Autodesk Inventor part; units mm, degrees
(part 2 of 2)
sketch "Sketch10" plane through (0, 5.08, 0) normal (0, 1, 0) x (1, 0, 0)
  line L0 (-146.4702, 23.2181) -> (-107.0908, 23.2181) construction
  line L1 (-107.0908, 23.2181) -> (-107.0908, 13.5732) construction
  line L2 (-107.0908, 13.5732) -> (-146.4702, 13.5732) construction
  line L3 (-146.4702, 13.5732) -> (-146.4702, 23.2181) construction
  spline S0 degree 2 poles (-138.3409, 21.7608) (-138.5381, 21.3498) (-139.1463, 19.9801) knots 0 0 0 1 1 1
  spline S1 degree 2 poles (-139.1463, 19.9801) (-139.6503, 18.8296) (-140.001, 18.1776) knots 0 0 0 1 1 1
  spline S2 degree 2 poles (-140.001, 18.1776) (-140.6146, 17.0489) (-140.6584, 16.9777) knots 0 0 0 1 1 1
  spline S3 degree 2 poles (-140.6584, 16.9777) (-140.8886, 16.638) (-141.1899, 16.638) knots 0 0 0 1 1 1
  spline S4 degree 2 poles (-141.1899, 16.638) (-141.409, 16.638) (-141.5734, 16.7805) knots 0 0 0 1 1 1
  spline S5 degree 2 poles (-141.5734, 16.7805) (-141.7542, 16.9394) (-141.7542, 17.1695) knots 0 0 0 1 1 1
  spline S6 degree 2 poles (-141.7542, 17.1695) (-141.7542, 17.3612) (-140.9324, 18.7857) knots 0 0 0 1 1 1
  spline S7 degree 2 poles (-140.9324, 18.7857) (-141.2337, 19.224) (-141.798, 20.1116) knots 0 0 0 1 1 1
  spline S8 degree 2 poles (-141.798, 20.1116) (-142.2254, 20.7636) (-143.0472, 22.0785) knots 0 0 0 1 1 1
  spline S9 degree 2 poles (-143.0472, 22.0785) (-143.1239, 22.2155) (-143.1239, 22.358) knots 0 0 0 1 1 1
  spline S10 degree 2 poles (-143.1239, 22.358) (-143.1239, 22.5881) (-142.9486, 22.7415) knots 0 0 0 1 1 1
  spline S11 degree 2 poles (-142.9486, 22.7415) (-142.7788, 22.8894) (-142.5596, 22.8894) knots 0 0 0 1 1 1
  spline S12 degree 2 poles (-142.5596, 22.8894) (-142.3021, 22.8894) (-142.0884, 22.6264) knots 0 0 0 1 1 1
  line L4 (-142.0884, 22.6264) -> (-141.7926, 22.1552)
  spline S13 degree 2 poles (-141.7926, 22.1552) (-141.7652, 22.1059) (-141.1187, 21.0047) knots 0 0 0 1 1 1
  spline S14 degree 2 poles (-141.1187, 21.0047) (-140.7132, 20.3034) (-140.4009, 19.8979) knots 0 0 0 1 1 1
  spline S15 degree 2 poles (-140.4009, 19.8979) (-140.0996, 20.4951) (-139.5408, 21.7169) knots 0 0 0 1 1 1
  spline S16 degree 2 poles (-139.5408, 21.7169) (-139.4202, 21.9854) (-139.1846, 22.5333) knots 0 0 0 1 1 1
  spline S17 degree 2 poles (-139.1846, 22.5333) (-139.0367, 22.8894) (-138.6751, 22.8894) knots 0 0 0 1 1 1
  spline S18 degree 2 poles (-138.6751, 22.8894) (-138.4559, 22.8894) (-138.2916, 22.747) knots 0 0 0 1 1 1
  spline S19 degree 2 poles (-138.2916, 22.747) (-138.1108, 22.5935) (-138.1108, 22.3634) knots 0 0 0 1 1 1
  spline S20 degree 2 poles (-138.1108, 22.3634) (-138.1108, 22.2319) (-138.3409, 21.7608) knots 0 0 0 1 1 1
  spline S21 degree 2 poles (-133.6126, 21.9525) (-133.6893, 21.9525) (-133.777, 21.9744) knots 0 0 0 1 1 1
  spline S22 degree 2 poles (-133.777, 21.9744) (-134.4125, 22.1443) (-135.0152, 22.1443) knots 0 0 0 1 1 1
  spline S23 degree 2 poles (-135.0152, 22.1443) (-135.3111, 22.1443) (-135.985, 22.0511) (-136.3685, 21.958) knots 0 0 0 1 2 2 2
  spline S24 degree 2 poles (-136.3685, 21.958) (-136.3685, 21.4375) (-136.4014, 20.4075) knots 0 0 0 1 1 1
  spline S25 degree 2 poles (-136.4014, 20.4075) (-136.1822, 20.4239) (-134.8618, 20.5499) knots 0 0 0 1 1 1
  spline S26 degree 2 poles (-134.8618, 20.5499) (-134.1112, 20.6266) (-133.914, 20.6266) knots 0 0 0 1 1 1
  spline S27 degree 2 poles (-133.914, 20.6266) (-133.6784, 20.6266) (-133.3496, 20.3308) (-133.3496, 20.0897) knots 0 0 0 1 2 2 2
  spline S28 degree 2 poles (-133.3496, 20.0897) (-133.3496, 19.6185) (-133.8482, 19.5583) knots 0 0 0 1 1 1
  spline S29 degree 2 poles (-133.8482, 19.5583) (-134.166, 19.5363) (-134.7906, 19.4816) knots 0 0 0 1 1 1
  spline S30 degree 2 poles (-134.7906, 19.4816) (-135.3494, 19.4158) (-136.4726, 19.3281) knots 0 0 0 1 1 1
  spline S31 degree 2 poles (-136.4726, 19.3281) (-136.5, 18.8296) (-136.5, 18.5228) knots 0 0 0 1 1 1
  spline S32 degree 2 poles (-136.5, 18.5228) (-136.5, 17.7448) (-136.4123, 17.6407) knots 0 0 0 1 1 1
  spline S33 degree 2 poles (-136.4123, 17.6407) (-136.3685, 17.5913) (-135.9137, 17.5913) knots 0 0 0 1 1 1
  spline S34 degree 2 poles (-135.9137, 17.5913) (-135.6727, 17.5913) (-134.6865, 17.6133) (-134.4399, 17.6133) knots 0 0 0 1 2 2 2
  spline S35 degree 2 poles (-134.4399, 17.6133) (-134.3632, 17.6133) (-134.0564, 17.6626) (-133.9797, 17.6626) knots 0 0 0 1 2 2 2
  spline S36 degree 2 poles (-133.9797, 17.6626) (-133.7496, 17.6626) (-133.5907, 17.5311) knots 0 0 0 1 1 1
  spline S37 degree 2 poles (-133.5907, 17.5311) (-133.4044, 17.3832) (-133.4044, 17.1256) knots 0 0 0 1 1 1
  spline S38 degree 2 poles (-133.4044, 17.1256) (-133.4044, 16.6819) (-133.8647, 16.5997) knots 0 0 0 1 1 1
  spline S39 degree 2 poles (-133.8647, 16.5997) (-134.2591, 16.523) (-135.4974, 16.523) knots 0 0 0 1 1 1
  spline S40 degree 2 poles (-135.4974, 16.523) (-136.7794, 16.523) (-137.1684, 16.8681) knots 0 0 0 1 1 1
  spline S41 degree 2 poles (-137.1684, 16.8681) (-137.5958, 17.2517) (-137.5958, 18.5228) knots 0 0 0 1 1 1
  spline S42 degree 2 poles (-137.5958, 18.5228) (-137.5958, 19.0487) (-137.4478, 21.1581) (-137.4478, 21.6786) knots 0 0 0 1 2 2 2
  spline S43 degree 2 poles (-137.4478, 21.6786) (-137.4478, 21.821) (-137.5245, 22.358) (-137.5245, 22.4949) knots 0 0 0 1 2 2 2
  spline S44 degree 2 poles (-137.5245, 22.4949) (-137.5245, 23.0921) (-136.9766, 23.0921) knots 0 0 0 1 1 1
  spline S45 degree 2 poles (-136.9766, 23.0921) (-136.8013, 23.0921) (-136.6589, 22.9935) knots 0 0 0 1 1 1
  spline S46 degree 2 poles (-136.6589, 22.9935) (-136.1987, 23.1086) (-135.3823, 23.2181) (-135.0152, 23.2181) knots 0 0 0 1 2 2 2
  spline S47 degree 2 poles (-135.0152, 23.2181) (-134.0235, 23.2181) (-133.4318, 22.9935) knots 0 0 0 1 1 1
  spline S48 degree 2 poles (-133.4318, 22.9935) (-133.0702, 22.8565) (-133.0702, 22.4949) knots 0 0 0 1 1 1
  spline S49 degree 2 poles (-133.0702, 22.4949) (-133.0702, 22.2922) (-133.2127, 22.1333) knots 0 0 0 1 1 1
  spline S50 degree 2 poles (-133.2127, 22.1333) (-133.3716, 21.9525) (-133.6126, 21.9525) knots 0 0 0 1 1 1
  spline S51 degree 2 poles (-130.6979, 16.6709) (-131.695, 16.6709) (-132.2703, 17.1147) knots 0 0 0 1 1 1
  spline S52 degree 2 poles (-132.2703, 17.1147) (-132.7524, 17.4818) (-132.7524, 17.9639) knots 0 0 0 1 1 1
  spline S53 degree 2 poles (-132.7524, 17.9639) (-132.7524, 18.2159) (-132.4566, 18.5392) (-132.1936, 18.5392) knots 0 0 0 1 2 2 2
  spline S54 degree 2 poles (-132.1936, 18.5392) (-131.8375, 18.5392) (-131.6731, 18.1776) knots 0 0 0 1 1 1
  spline S55 degree 2 poles (-131.6731, 18.1776) (-131.4485, 17.6954) (-130.6595, 17.6954) knots 0 0 0 1 1 1
  spline S56 degree 2 poles (-130.6595, 17.6954) (-129.9801, 17.6954) (-129.3501, 17.9913) knots 0 0 0 1 1 1
  spline S57 degree 2 poles (-129.3501, 17.9913) (-128.6926, 18.2926) (-128.6926, 18.6542) knots 0 0 0 1 1 1
  spline S58 degree 2 poles (-128.6926, 18.6542) (-128.6926, 19.1528) (-129.1035, 19.3117) knots 0 0 0 1 1 1
  spline S59 degree 2 poles (-129.1035, 19.3117) (-129.3939, 19.4213) (-130.2705, 19.4432) knots 0 0 0 1 1 1
  spline S60 degree 2 poles (-130.2705, 19.4432) (-130.9499, 19.4596) (-131.4868, 19.7007) knots 0 0 0 1 1 1
  spline S61 degree 2 poles (-131.4868, 19.7007) (-132.2155, 20.024) (-132.2046, 20.6321) knots 0 0 0 1 1 1
  spline S62 degree 2 poles (-132.2046, 20.6321) (-132.1936, 21.3992) (-130.5828, 22.6757) (-129.6076, 22.6757) knots 0 0 0 1 2 2 2
  spline S63 degree 2 poles (-129.6076, 22.6757) (-129.2241, 22.6757) (-128.6543, 22.5004) knots 0 0 0 1 1 1
  spline S64 degree 2 poles (-128.6543, 22.5004) (-127.953, 22.2813) (-127.953, 21.9909) knots 0 0 0 1 1 1
  spline S65 degree 2 poles (-127.953, 21.9909) (-127.953, 21.7882) (-128.0954, 21.6293) knots 0 0 0 1 1 1
  spline S66 degree 2 poles (-128.0954, 21.6293) (-128.2543, 21.4539) (-128.5009, 21.4539) knots 0 0 0 1 1 1
  spline S67 degree 2 poles (-128.5009, 21.4539) (-128.6817, 21.4539) (-129.4213, 21.6128) (-129.6076, 21.6128) knots 0 0 0 1 2 2 2
  spline S68 degree 2 poles (-129.6076, 21.6128) (-130.1171, 21.6074) (-130.5719, 21.3718) knots 0 0 0 1 1 1
  spline S69 degree 2 poles (-130.5719, 21.3718) (-131.043, 21.1252) (-131.043, 20.8403) knots 0 0 0 1 1 1
  spline S70 degree 2 poles (-131.043, 20.8403) (-131.043, 20.6869) (-130.7581, 20.4951) (-130.4678, 20.4568) knots 0 0 0 1 2 2 2
  spline S71 degree 2 poles (-130.4678, 20.4568) (-129.9692, 20.4294) (-129.4651, 20.402) knots 0 0 0 1 1 1
  spline S72 degree 2 poles (-129.4651, 20.402) (-128.594, 20.3363) (-128.0899, 19.9089) knots 0 0 0 1 1 1
  spline S73 degree 2 poles (-128.0899, 19.9089) (-127.5311, 19.4377) (-127.5311, 18.6049) knots 0 0 0 1 1 1
  spline S74 degree 2 poles (-127.5311, 18.6049) (-127.5311, 17.5913) (-128.6871, 17.0654) knots 0 0 0 1 1 1
  spline S75 degree 2 poles (-128.6871, 17.0654) (-129.5638, 16.6709) (-130.6979, 16.6709) knots 0 0 0 1 1 1
  spline S76 degree 2 poles (-115.8063, 21.9525) (-115.8721, 21.7936) (-115.9652, 21.558) knots 0 0 0 1 1 1
  spline S77 degree 2 poles (-115.9652, 21.558) (-116.031, 21.3279) (-116.1789, 20.8841) knots 0 0 0 1 1 1
  spline S78 degree 2 poles (-116.1789, 20.8841) (-116.4035, 20.3034) (-116.8911, 19.1967) knots 0 0 0 1 1 1
  spline S79 degree 2 poles (-116.8911, 19.1967) (-117.3897, 18.0735) (-117.6089, 17.5201) knots 0 0 0 1 1 1
  spline S80 degree 2 poles (-117.6089, 17.5201) (-117.7678, 17.1092) (-117.9102, 16.8627) knots 0 0 0 1 1 1
  spline S81 degree 2 poles (-117.9102, 16.8627) (-118.0965, 16.5339) (-118.4745, 16.5339) knots 0 0 0 1 1 1
  spline S82 degree 2 poles (-118.4745, 16.5339) (-118.6937, 16.5339) (-118.8745, 16.6545) knots 0 0 0 1 1 1
  spline S83 degree 2 poles (-118.8745, 16.6545) (-119.0882, 16.7969) (-119.1046, 17.027) knots 0 0 0 1 1 1
  spline S84 degree 2 poles (-119.1046, 17.027) (-119.2854, 17.4818) (-119.3347, 17.7667) knots 0 0 0 1 1 1
  spline S85 degree 2 poles (-119.3347, 17.7667) (-119.5046, 18.6104) (-119.8114, 20.2979) knots 0 0 0 1 1 1
  spline S86 degree 2 poles (-119.8114, 20.2979) (-120.0689, 19.5035) (-120.3647, 18.8789) knots 0 0 0 1 1 1
  spline S87 degree 2 poles (-120.3647, 18.8789) (-120.8031, 17.931) (-120.94, 17.3941) knots 0 0 0 1 1 1
  spline S88 degree 2 poles (-120.94, 17.3941) (-120.9071, 17.3064) (-120.9071, 17.2078) knots 0 0 0 1 1 1
  spline S89 degree 2 poles (-120.9071, 17.2078) (-120.9071, 16.9668) (-121.1208, 16.8133) knots 0 0 0 1 1 1
  spline S90 degree 2 poles (-121.1208, 16.8133) (-121.3126, 16.6819) (-121.5372, 16.6819) knots 0 0 0 1 1 1
  spline S91 degree 2 poles (-121.5372, 16.6819) (-121.8276, 16.6819) (-122.0139, 16.8298) knots 0 0 0 1 1 1
  spline S92 degree 2 poles (-122.0139, 16.8298) (-122.2221, 16.9887) (-122.2276, 17.2681) knots 0 0 0 1 1 1
  line L5 (-122.2276, 17.2681) -> (-122.3481, 17.7283)
  spline S93 degree 2 poles (-122.3481, 17.7283) (-122.4796, 18.342) (-122.7754, 19.5583) knots 0 0 0 1 1 1
  spline S94 degree 2 poles (-122.7754, 19.5583) (-123.0329, 20.4951) (-123.6466, 22.2155) knots 0 0 0 1 1 1
  spline S95 degree 2 poles (-123.6466, 22.2155) (-123.6795, 22.3141) (-123.6795, 22.4127) knots 0 0 0 1 1 1
  spline S96 degree 2 poles (-123.6795, 22.4127) (-123.6795, 22.6483) (-123.4987, 22.7853) knots 0 0 0 1 1 1
  spline S97 degree 2 poles (-123.4987, 22.7853) (-123.3398, 22.9113) (-123.1097, 22.9113) knots 0 0 0 1 1 1
  spline S98 degree 2 poles (-123.1097, 22.9113) (-122.8083, 22.9113) (-122.633, 22.6593) knots 0 0 0 1 1 1
  spline S99 degree 2 poles (-122.633, 22.6593) (-122.5344, 22.5223) (-122.4084, 22.1607) knots 0 0 0 1 1 1
  spline S100 degree 2 poles (-122.4084, 22.1607) (-122.0248, 21.0485) (-121.5372, 18.9282) knots 0 0 0 1 1 1
  spline S101 degree 2 poles (-121.5372, 18.9282) (-121.2249, 19.6952) (-120.8962, 20.7362) knots 0 0 0 1 1 1
  spline S102 degree 2 poles (-120.8962, 20.7362) (-120.6332, 21.5854) (-120.4688, 21.947) knots 0 0 0 1 1 1
  spline S103 degree 2 poles (-120.4688, 21.947) (-120.0744, 22.8017) (-119.6689, 22.8017) knots 0 0 0 1 1 1
  spline S104 degree 2 poles (-119.6689, 22.8017) (-119.2799, 22.8017) (-119.1046, 22.3799) knots 0 0 0 1 1 1
  spline S105 degree 2 poles (-119.1046, 22.3799) (-119.0169, 22.1826) (-118.9348, 21.6512) knots 0 0 0 1 1 1
  spline S106 degree 2 poles (-118.9348, 21.6512) (-118.9128, 21.4923) (-118.8361, 20.8622) knots 0 0 0 1 1 1
  spline S107 degree 2 poles (-118.8361, 20.8622) (-118.7485, 20.1883) (-118.3376, 18.4022) knots 0 0 0 1 1 1
  spline S108 degree 2 poles (-118.3376, 18.4022) (-117.9212, 19.3775) (-117.2199, 21.2129) knots 0 0 0 1 1 1
  spline S109 degree 2 poles (-117.2199, 21.2129) (-117.176, 21.3225) (-117.0117, 21.9361) knots 0 0 0 1 1 1
  spline S110 degree 2 poles (-117.0117, 21.9361) (-116.9021, 22.3744) (-116.7268, 22.6319) knots 0 0 0 1 1 1
  spline S111 degree 2 poles (-116.7268, 22.6319) (-116.5405, 22.9058) (-116.2227, 22.9058) knots 0 0 0 1 1 1
  spline S112 degree 2 poles (-116.2227, 22.9058) (-115.9817, 22.9058) (-115.6694, 22.61) (-115.6694, 22.3799) knots 0 0 0 1 2 2 2
  spline S113 degree 2 poles (-115.6694, 22.3799) (-115.6694, 22.2977) (-115.8063, 21.9525) knots 0 0 0 1 1 1
  spline S114 degree 2 poles (-111.1493, 21.9525) (-111.226, 21.9525) (-111.3137, 21.9744) knots 0 0 0 1 1 1
  spline S115 degree 2 poles (-111.3137, 21.9744) (-111.9492, 22.1443) (-112.5519, 22.1443) knots 0 0 0 1 1 1
  spline S116 degree 2 poles (-112.5519, 22.1443) (-112.8477, 22.1443) (-113.5216, 22.0511) (-113.9052, 21.958) knots 0 0 0 1 2 2 2
  spline S117 degree 2 poles (-113.9052, 21.958) (-113.9052, 21.4375) (-113.938, 20.4075) knots 0 0 0 1 1 1
  spline S118 degree 2 poles (-113.938, 20.4075) (-113.7189, 20.4239) (-112.3985, 20.5499) knots 0 0 0 1 1 1
  spline S119 degree 2 poles (-112.3985, 20.5499) (-111.6479, 20.6266) (-111.4506, 20.6266) knots 0 0 0 1 1 1
  spline S120 degree 2 poles (-111.4506, 20.6266) (-111.215, 20.6266) (-110.8863, 20.3308) (-110.8863, 20.0897) knots 0 0 0 1 2 2 2
  spline S121 degree 2 poles (-110.8863, 20.0897) (-110.8863, 19.6185) (-111.3849, 19.5583) knots 0 0 0 1 1 1
  spline S122 degree 2 poles (-111.3849, 19.5583) (-111.7027, 19.5363) (-112.3273, 19.4816) knots 0 0 0 1 1 1
  spline S123 degree 2 poles (-112.3273, 19.4816) (-112.8861, 19.4158) (-114.0093, 19.3281) knots 0 0 0 1 1 1
  spline S124 degree 2 poles (-114.0093, 19.3281) (-114.0367, 18.8296) (-114.0367, 18.5228) knots 0 0 0 1 1 1
  spline S125 degree 2 poles (-114.0367, 18.5228) (-114.0367, 17.7448) (-113.949, 17.6407) knots 0 0 0 1 1 1
  spline S126 degree 2 poles (-113.949, 17.6407) (-113.9052, 17.5913) (-113.4504, 17.5913) knots 0 0 0 1 1 1
  spline S127 degree 2 poles (-113.4504, 17.5913) (-113.2093, 17.5913) (-112.2232, 17.6133) (-111.9766, 17.6133) knots 0 0 0 1 2 2 2
  spline S128 degree 2 poles (-111.9766, 17.6133) (-111.8999, 17.6133) (-111.5931, 17.6626) (-111.5164, 17.6626) knots 0 0 0 1 2 2 2
  spline S129 degree 2 poles (-111.5164, 17.6626) (-111.2863, 17.6626) (-111.1274, 17.5311) knots 0 0 0 1 1 1
  spline S130 degree 2 poles (-111.1274, 17.5311) (-110.9411, 17.3832) (-110.9411, 17.1256) knots 0 0 0 1 1 1
  spline S131 degree 2 poles (-110.9411, 17.1256) (-110.9411, 16.6819) (-111.4013, 16.5997) knots 0 0 0 1 1 1
  spline S132 degree 2 poles (-111.4013, 16.5997) (-111.7958, 16.523) (-113.034, 16.523) knots 0 0 0 1 1 1
  spline S133 degree 2 poles (-113.034, 16.523) (-114.3161, 16.523) (-114.7051, 16.8681) knots 0 0 0 1 1 1
  spline S134 degree 2 poles (-114.7051, 16.8681) (-115.1324, 17.2517) (-115.1324, 18.5228) knots 0 0 0 1 1 1
  spline S135 degree 2 poles (-115.1324, 18.5228) (-115.1324, 19.0487) (-114.9845, 21.1581) (-114.9845, 21.6786) knots 0 0 0 1 2 2 2
  spline S136 degree 2 poles (-114.9845, 21.6786) (-114.9845, 21.821) (-115.0612, 22.358) (-115.0612, 22.4949) knots 0 0 0 1 2 2 2
  spline S137 degree 2 poles (-115.0612, 22.4949) (-115.0612, 23.0921) (-114.5133, 23.0921) knots 0 0 0 1 1 1
  spline S138 degree 2 poles (-114.5133, 23.0921) (-114.338, 23.0921) (-114.1955, 22.9935) knots 0 0 0 1 1 1
  spline S139 degree 2 poles (-114.1955, 22.9935) (-113.7353, 23.1086) (-112.919, 23.2181) (-112.5519, 23.2181) knots 0 0 0 1 2 2 2
  spline S140 degree 2 poles (-112.5519, 23.2181) (-111.5602, 23.2181) (-110.9685, 22.9935) knots 0 0 0 1 1 1
  spline S141 degree 2 poles (-110.9685, 22.9935) (-110.6069, 22.8565) (-110.6069, 22.4949) knots 0 0 0 1 1 1
  spline S142 degree 2 poles (-110.6069, 22.4949) (-110.6069, 22.2922) (-110.7493, 22.1333) knots 0 0 0 1 1 1
  spline S143 degree 2 poles (-110.7493, 22.1333) (-110.9082, 21.9525) (-111.1493, 21.9525) knots 0 0 0 1 1 1
  spline S144 degree 2 poles (-134.4153, 7.617) (-134.7659, 7.617) (-134.9358, 7.9896) knots 0 0 0 1 1 1
  spline S145 degree 2 poles (-134.9358, 7.9896) (-135.0125, 8.1704) (-135.0947, 8.2033) knots 0 0 0 1 1 1
  spline S146 degree 2 poles (-135.0947, 8.2033) (-135.1549, 8.2307) (-135.407, 8.2307) knots 0 0 0 1 1 1
  spline S147 degree 2 poles (-135.407, 8.2307) (-135.9001, 8.2307) (-136.5466, 7.4581) knots 0 0 0 1 1 1
  spline S148 degree 2 poles (-136.5466, 7.4581) (-137.456, 6.3843) (-137.456, 5.4419) knots 0 0 0 1 1 1
  spline S149 degree 2 poles (-137.456, 5.4419) (-137.456, 5.0146) (-136.8808, 4.4009) (-136.4808, 4.4009) knots 0 0 0 1 2 2 2
  spline S150 degree 2 poles (-136.4808, 4.4009) (-136.0918, 4.4009) (-135.6919, 4.6037) knots 0 0 0 1 1 1
  spline S151 degree 2 poles (-135.6919, 4.6037) (-135.5494, 4.6804) (-135.0947, 4.9927) knots 0 0 0 1 1 1
  spline S152 degree 2 poles (-135.0947, 4.9927) (-134.7878, 5.1954) (-134.629, 5.1954) knots 0 0 0 1 1 1
  spline S153 degree 2 poles (-134.629, 5.1954) (-134.3934, 5.1954) (-134.229, 5.0201) knots 0 0 0 1 1 1
  spline S154 degree 2 poles (-134.229, 5.0201) (-134.0756, 4.8612) (-134.0756, 4.653) knots 0 0 0 1 1 1
  spline S155 degree 2 poles (-134.0756, 4.653) (-134.0756, 4.4229) (-134.2783, 4.2475) knots 0 0 0 1 1 1
  spline S156 degree 2 poles (-134.2783, 4.2475) (-135.3631, 3.338) (-136.4808, 3.338) knots 0 0 0 1 1 1
  spline S157 degree 2 poles (-136.4808, 3.338) (-137.3684, 3.338) (-137.9765, 3.9845) knots 0 0 0 1 1 1
  spline S158 degree 2 poles (-137.9765, 3.9845) (-138.5573, 4.6037) (-138.5573, 5.4419) knots 0 0 0 1 1 1
  spline S159 degree 2 poles (-138.5573, 5.4419) (-138.5573, 6.7623) (-137.4067, 8.132) knots 0 0 0 1 1 1
  spline S160 degree 2 poles (-137.4067, 8.132) (-136.426, 9.2936) (-135.407, 9.2936) knots 0 0 0 1 1 1
  spline S161 degree 2 poles (-135.407, 9.2936) (-135.2316, 9.2936) (-134.9522, 9.2716) (-134.8481, 9.2443) knots 0 0 0 1 2 2 2
  spline S162 degree 2 poles (-134.8481, 9.2443) (-134.6728, 9.4141) (-134.4317, 9.4141) knots 0 0 0 1 1 1
  spline S163 degree 2 poles (-134.4317, 9.4141) (-134.0263, 9.4141) (-133.9331, 8.9539) knots 0 0 0 1 1 1
  spline S164 degree 2 poles (-133.9331, 8.9539) (-133.8674, 8.6251) (-133.8674, 8.1868) knots 0 0 0 1 1 1
  spline S165 degree 2 poles (-133.8674, 8.1868) (-133.8674, 7.9896) (-133.9825, 7.8307) knots 0 0 0 1 1 1
  spline S166 degree 2 poles (-133.9825, 7.8307) (-134.1304, 7.617) (-134.4153, 7.617) knots 0 0 0 1 1 1
  spline S167 degree 2 poles (-128.8652, 3.3106) (-129.1775, 3.3216) (-129.4898, 4.0448) knots 0 0 0 1 1 1
  spline S168 degree 2 poles (-129.4898, 4.0448) (-129.698, 4.505) (-129.8459, 5.1132) knots 0 0 0 1 1 1
  spline S169 degree 2 poles (-129.8459, 5.1132) (-130.1363, 5.0694) (-130.7992, 5.0255) knots 0 0 0 1 1 1
  spline S170 degree 2 poles (-130.7992, 5.0255) (-131.4183, 4.9872) (-131.7471, 4.9269) knots 0 0 0 1 1 1
  spline S171 degree 2 poles (-131.7471, 4.9269) (-131.9279, 4.4941) (-132.3771, 3.6229) knots 0 0 0 1 1 1
  spline S172 degree 2 poles (-132.3771, 3.6229) (-132.5525, 3.338) (-132.8538, 3.338) knots 0 0 0 1 1 1
  spline S173 degree 2 poles (-132.8538, 3.338) (-133.073, 3.338) (-133.4181, 3.6339) (-133.4181, 3.8585) knots 0 0 0 1 2 2 2
  spline S174 degree 2 poles (-133.4181, 3.8585) (-133.4181, 4.0613) (-132.8428, 5.2228) knots 0 0 0 1 1 1
  spline S175 degree 2 poles (-132.8428, 5.2228) (-132.8976, 5.3433) (-132.8922, 5.4474) knots 0 0 0 1 1 1
  spline S176 degree 2 poles (-132.8922, 5.4474) (-132.8757, 5.6392) (-132.5086, 5.7433) knots 0 0 0 1 1 1
  spline S177 degree 2 poles (-132.5086, 5.7433) (-131.9498, 6.713) (-131.2649, 7.7485) knots 0 0 0 1 1 1
  spline S178 degree 2 poles (-131.2649, 7.7485) (-130.2842, 9.2388) (-130.0541, 9.2388) knots 0 0 0 1 1 1
  spline S179 degree 2 poles (-130.0541, 9.2388) (-129.6268, 9.2388) (-129.4788, 8.7183) knots 0 0 0 1 1 1
  spline S180 degree 2 poles (-129.4788, 8.7183) (-129.4021, 8.2964) (-129.2323, 7.4527) knots 0 0 0 1 1 1
  spline S181 degree 2 poles (-129.2323, 7.4527) (-128.9912, 6.324) (-128.646, 4.8612) knots 0 0 0 1 1 1
  spline S182 degree 2 poles (-128.646, 4.8612) (-128.6186, 4.7516) (-128.4488, 4.3462) knots 0 0 0 1 1 1
  spline S183 degree 2 poles (-128.4488, 4.3462) (-128.3064, 4.0065) (-128.3064, 3.8366) knots 0 0 0 1 1 1
  spline S184 degree 2 poles (-128.3064, 3.8366) (-128.3064, 3.612) (-128.646, 3.3052) (-128.8652, 3.3106) knots 0 0 0 1 2 2 2
  spline S185 degree 2 poles (-130.3281, 7.3431) (-130.6349, 6.8171) (-131.1718, 5.9131) knots 0 0 0 1 1 1
  spline S186 degree 2 poles (-131.1718, 5.9131) (-130.9965, 5.9515) (-130.6239, 5.9734) knots 0 0 0 1 1 1
  spline S187 degree 2 poles (-130.6239, 5.9734) (-130.1801, 6.0008) (-130.0705, 6.0172) knots 0 0 0 1 1 1
  spline S188 degree 2 poles (-130.0705, 6.0172) (-130.1637, 6.5267) (-130.3281, 7.3431) knots 0 0 0 1 1 1
  spline S189 degree 2 poles (-121.6769, 4.4009) (-121.6769, 4.2037) (-121.7427, 3.7818) knots 0 0 0 1 1 1
  spline S190 degree 2 poles (-121.7427, 3.7818) (-121.8249, 3.2723) (-122.318, 3.2723) knots 0 0 0 1 1 1
  spline S191 degree 2 poles (-122.318, 3.2723) (-122.5919, 3.2723) (-122.9425, 3.5846) knots 0 0 0 1 1 1
  spline S192 degree 2 poles (-122.9425, 3.5846) (-124.4547, 4.9488) (-126.3559, 7.4088) knots 0 0 0 1 1 1
  spline S193 degree 2 poles (-126.3559, 7.4088) (-126.3778, 6.3843) (-126.3778, 6.1542) knots 0 0 0 1 1 1
  spline S194 degree 2 poles (-126.3778, 6.1542) (-126.3778, 5.8419) (-126.3504, 4.5927) (-126.3504, 4.2859) knots 0 0 0 1 2 2 2
  spline S195 degree 2 poles (-126.3504, 4.2859) (-126.3504, 3.1244) (-126.9147, 3.1244) knots 0 0 0 1 1 1
  spline S196 degree 2 poles (-126.9147, 3.1244) (-127.2051, 3.1244) (-127.3749, 3.2997) knots 0 0 0 1 1 1
  spline S197 degree 2 poles (-127.3749, 3.2997) (-127.5284, 3.4586) (-127.5284, 3.6832) knots 0 0 0 1 1 1
  spline S198 degree 2 poles (-127.5284, 3.6832) (-127.5284, 3.8421) (-127.479, 4.4776) (-127.479, 4.6311) knots 0 0 0 1 2 2 2
  spline S199 degree 2 poles (-127.479, 4.6311) (-127.479, 4.8666) (-127.4462, 5.7926) (-127.4462, 6.0227) knots 0 0 0 1 2 2 2
  spline S200 degree 2 poles (-127.4462, 6.0227) (-127.4462, 6.2692) (-127.4681, 7.2719) (-127.4681, 7.5184) knots 0 0 0 1 2 2 2
  spline S201 degree 2 poles (-127.4681, 7.5184) (-127.4681, 7.754) (-127.5612, 8.6909) (-127.5612, 8.9265) knots 0 0 0 1 2 2 2
  spline S202 degree 2 poles (-127.5612, 8.9265) (-127.5612, 9.1621) (-127.1558, 9.5292) (-126.8983, 9.5292) knots 0 0 0 1 2 2 2
  spline S203 degree 2 poles (-126.8983, 9.5292) (-126.6079, 9.5292) (-126.2518, 9.0251) knots 0 0 0 1 1 1
  spline S204 degree 2 poles (-126.2518, 9.0251) (-124.4711, 6.4774) (-122.7343, 4.8721) knots 0 0 0 1 1 1
  spline S205 degree 2 poles (-122.7343, 4.8721) (-122.7289, 4.9981) (-122.7289, 5.4693) knots 0 0 0 1 1 1
  spline S206 degree 2 poles (-122.7289, 5.4693) (-122.7289, 7.4034) (-122.7672, 8.0827) knots 0 0 0 1 1 1
  spline S207 degree 2 poles (-122.7672, 8.0827) (-122.7782, 8.1978) (-122.8165, 8.5046) knots 0 0 0 1 1 1
  spline S208 degree 2 poles (-122.8165, 8.5046) (-122.8549, 8.7785) (-122.8549, 8.9374) knots 0 0 0 1 1 1
  spline S209 degree 2 poles (-122.8549, 8.9374) (-122.8549, 9.4798) (-122.2851, 9.4798) knots 0 0 0 1 1 1
  spline S210 degree 2 poles (-122.2851, 9.4798) (-121.6495, 9.4798) (-121.6495, 7.502) knots 0 0 0 1 1 1
  spline S211 degree 2 poles (-121.6495, 7.502) (-121.6495, 7.4581) (-121.655, 6.8829) knots 0 0 0 1 1 1
  spline S212 degree 2 poles (-121.655, 6.8829) (-121.6769, 4.8886) (-121.6769, 4.4009) knots 0 0 0 1 1 1
  spline S213 degree 2 poles (-115.1352, 4.4009) (-115.1352, 4.2037) (-115.2009, 3.7818) knots 0 0 0 1 1 1
  spline S214 degree 2 poles (-115.2009, 3.7818) (-115.2831, 3.2723) (-115.7762, 3.2723) knots 0 0 0 1 1 1
  spline S215 degree 2 poles (-115.7762, 3.2723) (-116.0501, 3.2723) (-116.4008, 3.5846) knots 0 0 0 1 1 1
  spline S216 degree 2 poles (-116.4008, 3.5846) (-117.913, 4.9488) (-119.8141, 7.4088) knots 0 0 0 1 1 1
  spline S217 degree 2 poles (-119.8141, 7.4088) (-119.836, 6.3843) (-119.836, 6.1542) knots 0 0 0 1 1 1
  spline S218 degree 2 poles (-119.836, 6.1542) (-119.836, 5.8419) (-119.8086, 4.5927) (-119.8086, 4.2859) knots 0 0 0 1 2 2 2
  spline S219 degree 2 poles (-119.8086, 4.2859) (-119.8086, 3.1244) (-120.373, 3.1244) knots 0 0 0 1 1 1
  spline S220 degree 2 poles (-120.373, 3.1244) (-120.6633, 3.1244) (-120.8332, 3.2997) knots 0 0 0 1 1 1
  spline S221 degree 2 poles (-120.8332, 3.2997) (-120.9866, 3.4586) (-120.9866, 3.6832) knots 0 0 0 1 1 1
  spline S222 degree 2 poles (-120.9866, 3.6832) (-120.9866, 3.8421) (-120.9373, 4.4776) (-120.9373, 4.6311) knots 0 0 0 1 2 2 2
  spline S223 degree 2 poles (-120.9373, 4.6311) (-120.9373, 4.8666) (-120.9044, 5.7926) (-120.9044, 6.0227) knots 0 0 0 1 2 2 2
  spline S224 degree 2 poles (-120.9044, 6.0227) (-120.9044, 6.2692) (-120.9263, 7.2719) (-120.9263, 7.5184) knots 0 0 0 1 2 2 2
  spline S225 degree 2 poles (-120.9263, 7.5184) (-120.9263, 7.754) (-121.0195, 8.6909) (-121.0195, 8.9265) knots 0 0 0 1 2 2 2
  spline S226 degree 2 poles (-121.0195, 8.9265) (-121.0195, 9.1621) (-120.614, 9.5292) (-120.3565, 9.5292) knots 0 0 0 1 2 2 2
  spline S227 degree 2 poles (-120.3565, 9.5292) (-120.0661, 9.5292) (-119.71, 9.0251) knots 0 0 0 1 1 1
  spline S228 degree 2 poles (-119.71, 9.0251) (-117.9294, 6.4774) (-116.1926, 4.8721) knots 0 0 0 1 1 1
  spline S229 degree 2 poles (-116.1926, 4.8721) (-116.1871, 4.9981) (-116.1871, 5.4693) knots 0 0 0 1 1 1
  spline S230 degree 2 poles (-116.1871, 5.4693) (-116.1871, 7.4034) (-116.2255, 8.0827) knots 0 0 0 1 1 1
  spline S231 degree 2 poles (-116.2255, 8.0827) (-116.2364, 8.1978) (-116.2748, 8.5046) knots 0 0 0 1 1 1
  spline S232 degree 2 poles (-116.2748, 8.5046) (-116.3131, 8.7785) (-116.3131, 8.9374) knots 0 0 0 1 1 1
  spline S233 degree 2 poles (-116.3131, 8.9374) (-116.3131, 9.4798) (-115.7433, 9.4798) knots 0 0 0 1 1 1
  spline S234 degree 2 poles (-115.7433, 9.4798) (-115.1078, 9.4798) (-115.1078, 7.502) knots 0 0 0 1 1 1
  spline S235 degree 2 poles (-115.1078, 7.502) (-115.1078, 7.4581) (-115.1133, 6.8829) knots 0 0 0 1 1 1
  spline S236 degree 2 poles (-115.1133, 6.8829) (-115.1352, 4.8886) (-115.1352, 4.4009) knots 0 0 0 1 1 1
  point P0 (0, 0)
  constraints: 2 other
extrude "Extrusion7" cut sketch "Sketch10" against normal up to next
sketch "Sketch11" plane through (0, 2.54, 0) normal (0, 1, 0) x (1, 0, 0)
  line L0 (-205.5505, 105.9927) -> (-15.0505, 105.9927) construction
  line L1 (-15.0505, 105.9927) -> (-15.0505, -35.5593) construction
  line L2 (-15.0505, -35.5593) -> (-205.5505, -35.5593) construction
  line L3 (-205.5505, -35.5593) -> (-205.5505, 105.9927) construction
  line L4 (-130.347, 80.7217) -> (-132.9251, 82.8674) construction
  line L5 (-132.9251, 82.8674) -> (-135.4112, 84.8564) construction
  line L6 (-135.4112, 84.8564) -> (-140.2178, 87.5911) construction
  line L7 (-140.2178, 87.5911) -> (-143.367, 88.0277) construction
  line L8 (-143.367, 88.0277) -> (-147.7592, 88.0277) construction
  line L9 (-147.7592, 88.0277) -> (-149.4166, 86.8255) construction
  line L10 (-149.4166, 86.8255) -> (-149.4166, 86.1276) construction
  line L11 (-149.4166, 86.1276) -> (-148.4122, 86.4439) construction
  line L12 (-148.4122, 86.4439) -> (-147.2079, 86.8255) construction
  line L13 (-147.2079, 86.8255) -> (-145.6386, 86.9548) construction
  line L14 (-145.6386, 86.9548) -> (-143.9112, 86.602) construction
  line L15 (-143.9112, 86.602) -> (-139.0114, 85.2917) construction
  line L16 (-139.0114, 85.2917) -> (-136.4292, 83.2678) construction
  line L17 (-136.4292, 83.2678) -> (-133.2188, 81.3136) construction
  line L18 (-133.2188, 81.3136) -> (-130.7063, 80.0225) construction
  line L19 (-130.7063, 80.0225) -> (-130.2929, 80.2407) construction
  line L20 (-130.2929, 80.2407) -> (-130.347, 80.7217) construction
  spline S0 degree 4 poles (-130.347, 80.7217) (-132.9251, 82.8674) (-135.4112, 84.8564) (-140.2178, 87.5911) (-143.367, 88.0277) (-147.7592, 88.0277) (-149.4166, 86.8255) (-149.4166, 86.1276) (-148.4122, 86.4439) (-147.2079, 86.8255) (-145.6386, 86.9548) (-143.9112, 86.602) (-139.0114, 85.2917) (-136.4292, 83.2678) (-133.2188, 81.3136) (-130.7063, 80.0225) (-130.2929, 80.2407) (-130.347, 80.7217) knots 1 1 1 1 1 2 3 4 5 6 7 8 9 10 11 12 13 14 15 15 15 15 15
  line L21 (-117.5474, 81.3136) -> (-117.5474, 83.4914) construction
  line L22 (-117.5474, 83.4914) -> (-117.326, 89.9278) construction
  line L23 (-117.326, 89.9278) -> (-116.7891, 91.9353) construction
  line L24 (-116.7891, 91.9353) -> (-115.3861, 92.9529) construction
  line L25 (-115.3861, 92.9529) -> (-113.2213, 92.9529) construction
  line L26 (-113.2213, 92.9529) -> (-112.1928, 92.1468) construction
  line L27 (-112.1928, 92.1468) -> (-112.1928, 90.8707) construction
  line L28 (-112.1928, 90.8707) -> (-112.1928, 89.4774) construction
  line L29 (-112.1928, 89.4774) -> (-112.9403, 89.3933) construction
  line L30 (-112.9403, 89.3933) -> (-113.9804, 89.9278) construction
  line L31 (-113.9804, 89.9278) -> (-114.7276, 89.9278) construction
  line L32 (-114.7276, 89.9278) -> (-115.2356, 88.9393) construction
  line L33 (-115.2356, 88.9393) -> (-116.0137, 87.4252) construction
  line L34 (-116.0137, 87.4252) -> (-115.8282, 85.7759) construction
  line L35 (-115.8282, 85.7759) -> (-115.8282, 83.8604) construction
  line L36 (-115.8282, 83.8604) -> (-115.8282, 82.2892) construction
  line L37 (-115.8282, 82.2892) -> (-115.8282, 80.7203) construction
  line L38 (-115.8282, 80.7203) -> (-116.4203, 80.4078) construction
  line L39 (-116.4203, 80.4078) -> (-117.1876, 80.0029) construction
  line L40 (-117.1876, 80.0029) -> (-117.2181, 80.2746) construction
  line L41 (-117.2181, 80.2746) -> (-117.3958, 80.8353) construction
  spline S1 degree 4 poles (-117.5474, 81.3136) (-117.5474, 83.4914) (-117.326, 89.9278) (-116.7891, 91.9353) (-115.3861, 92.9529) (-113.2213, 92.9529) (-112.1928, 92.1468) (-112.1928, 90.8707) (-112.1928, 89.4774) (-112.9403, 89.3933) (-113.9804, 89.9278) (-114.7276, 89.9278) (-115.2356, 88.9393) (-116.0137, 87.4252) (-115.8282, 85.7759) (-115.8282, 83.8604) (-115.8282, 82.2892) (-115.8282, 80.7203) (-116.4203, 80.4078) (-117.1876, 80.0029) (-117.2181, 80.2746) (-117.3958, 80.8353) knots 1 1 1 1 1 2 3 4 5 6 7 8 9 10 11 12 13 14 15 16 17 18 19 19 19 19 19
  line L42 (-117.5474, 81.3136) -> (-117.3958, 80.8353) construction
  spline S2 degree 1 poles (-117.5474, 81.3136) (-117.3958, 80.8353) knots 1 1 2 2
  point P0 (-100.2607, 79.2979)
  point P1 (-112.1882, 86.8255)
  point P2 (-139.7824, 80.7529)
  point P3 (0, 0)
  constraints: 17 parallel, 5 perpendicular, 1 collinear, 10 other
extrude "Extrusion8" add sketch "Sketch11" along normal blind 2.54
sketch "Sketch12" plane through (0, 2.54, 0) normal (0, 1, 0) x (1, 0, 0)
  line L0 (-117.3958, 80.8353) -> (-117.5474, 81.3136) projected
  line L1 (-205.0821, 105.6604) -> (-14.5821, 105.6604) construction
  line L2 (-14.5821, 105.6604) -> (-14.5821, -35.8917) construction
  line L3 (-14.5821, -35.8917) -> (-205.0821, -35.8917) construction
  line L4 (-205.0821, -35.8917) -> (-205.0821, 105.6604) construction
  line L5 (-175.4731, 62.6944) -> (-173.1372, 61.0127) construction
  line L6 (-173.1372, 61.0127) -> (-169.8204, 58.6972) construction
  line L7 (-169.8204, 58.6972) -> (-168.0055, 56.4443) construction
  line L8 (-168.0055, 56.4443) -> (-166.8046, 56.0661) construction
  line L9 (-166.8046, 56.0661) -> (-165.6544, 56.4306) construction
  line L10 (-165.6544, 56.4306) -> (-165.2165, 57.3206) construction
  line L11 (-165.2165, 57.3206) -> (-165.972, 58.5421) construction
  line L12 (-165.972, 58.5421) -> (-168.4479, 60.5889) construction
  line L13 (-168.4479, 60.5889) -> (-171.1466, 61.5942) construction
  line L14 (-171.1466, 61.5942) -> (-174.4809, 62.4856) construction
  line L15 (-174.4809, 62.4856) -> (-175.4731, 62.6944) construction
  spline S0 degree 4 poles (-175.4731, 62.6944) (-173.1372, 61.0127) (-169.8204, 58.6972) (-168.0055, 56.4443) (-166.8046, 56.0661) (-165.6544, 56.4306) (-165.2165, 57.3206) (-165.972, 58.5421) (-168.4479, 60.5889) (-171.1466, 61.5942) (-174.4809, 62.4856) (-175.4731, 62.6944) knots 1 1 1 1 1 2 3 4 5 6 7 8 9 9 9 9 9
  line L16 (-179.2677, 56.9725) -> (-176.8648, 56.0825) construction
  line L17 (-176.8648, 56.0825) -> (-174.4307, 54.8054) construction
  line L18 (-174.4307, 54.8054) -> (-172.2678, 53.9996) construction
  line L19 (-172.2678, 53.9996) -> (-171.4788, 52.724) construction
  line L20 (-171.4788, 52.724) -> (-170.831, 51.6767) construction
  line L21 (-170.831, 51.6767) -> (-171.1466, 50.8296) construction
  line L22 (-171.1466, 50.8296) -> (-172.0438, 50.2747) construction
  line L23 (-172.0438, 50.2747) -> (-173.1372, 50.2747) construction
  line L24 (-173.1372, 50.2747) -> (-173.8176, 51.3748) construction
  line L25 (-173.8176, 51.3748) -> (-174.7886, 52.9448) construction
  line L26 (-174.7886, 52.9448) -> (-176.7249, 54.5454) construction
  line L27 (-176.7249, 54.5454) -> (-178.3638, 55.9002) construction
  line L28 (-178.3638, 55.9002) -> (-179.6387, 56.5275) construction
  line L29 (-179.6387, 56.5275) -> (-179.9452, 56.7809) construction
  line L30 (-179.9452, 56.7809) -> (-179.3406, 56.9725) construction
  line L31 (-179.3406, 56.9725) -> (-179.2677, 56.9725) construction
  spline S1 degree 4 poles (-179.2677, 56.9725) (-176.8648, 56.0825) (-174.4307, 54.8054) (-172.2678, 53.9996) (-171.4788, 52.724) (-170.831, 51.6767) (-171.1466, 50.8296) (-172.0438, 50.2747) (-173.1372, 50.2747) (-173.8176, 51.3748) (-174.7886, 52.9448) (-176.7249, 54.5454) (-178.3638, 55.9002) (-179.6387, 56.5275) (-179.9452, 56.7809) (-179.3406, 56.9725) (-179.2677, 56.9725) knots 1 1 1 1 1 2 3 4 5 6 7 8 9 10 11 12 13 14 14 14 14 14
  line L32 (-183.4415, 51.8181) -> (-181.0386, 50.9282) construction
  line L33 (-181.0386, 50.9282) -> (-178.6046, 49.6511) construction
  line L34 (-178.6046, 49.6511) -> (-176.4416, 48.8453) construction
  line L35 (-176.4416, 48.8453) -> (-175.6526, 47.5697) construction
  line L36 (-175.6526, 47.5697) -> (-175.0049, 46.5223) construction
  line L37 (-175.0049, 46.5223) -> (-175.3204, 45.6753) construction
  line L38 (-175.3204, 45.6753) -> (-176.2177, 45.1204) construction
  line L39 (-176.2177, 45.1204) -> (-177.311, 45.1204) construction
  line L40 (-177.311, 45.1204) -> (-177.9914, 46.2205) construction
  line L41 (-177.9914, 46.2205) -> (-178.9624, 47.7905) construction
  line L42 (-178.9624, 47.7905) -> (-180.8987, 49.3911) construction
  line L43 (-180.8987, 49.3911) -> (-182.5376, 50.7459) construction
  line L44 (-182.5376, 50.7459) -> (-183.8125, 51.3732) construction
  line L45 (-183.8125, 51.3732) -> (-184.119, 51.6265) construction
  line L46 (-184.119, 51.6265) -> (-183.5144, 51.8181) construction
  line L47 (-183.5144, 51.8181) -> (-183.4415, 51.8181) construction
  spline S2 degree 4 poles (-183.4415, 51.8181) (-181.0386, 50.9282) (-178.6046, 49.6511) (-176.4416, 48.8453) (-175.6526, 47.5697) (-175.0049, 46.5223) (-175.3204, 45.6753) (-176.2177, 45.1204) (-177.311, 45.1204) (-177.9914, 46.2205) (-178.9624, 47.7905) (-180.8987, 49.3911) (-182.5376, 50.7459) (-183.8125, 51.3732) (-184.119, 51.6265) (-183.5144, 51.8181) (-183.4415, 51.8181) knots 1 1 1 1 1 2 3 4 5 6 7 8 9 10 11 12 13 14 14 14 14 14
  point P0 (-130.347, 80.7217)
  point P1 (-100.2607, 79.2979)
  point P2 (-112.1882, 86.8255)
  point P3 (-139.7824, 80.7529)
  point P4 (0, 0)
  constraints: 9 parallel, 6 perpendicular, 8 other
extrude "Extrusion9" add sketch "Sketch12" along normal blind 2.54
body "Solid1"
